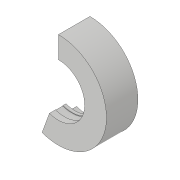
# Autodesk Inventor part: 00_Adapter_M8_Fluorescentfilter_Cellphone
Saved by Autodesk Inventor 2019 (Build 230136000, 136)
## iProperties
Created: 2019-06-13
Part Number: 00_Adapter_M8_Fluorescentfilter_Cellphone
Material: Generic
Document SubType Name: Modeling
Designer: diederichbenedict
Density: 1 g/cm^3
Appearance: Default
Author: diederichbenedict
Autodesk Inventor part; units mm, degrees
ref_plane "YZ Plane" through (0, 0, 0) normal (1, 0, 0) x (0, 1, 0)
ref_plane "XZ Plane" through (0, 0, 0) normal (0, 1, 0) x (-1, 0, 0)
ref_plane "XY Plane" through (0, 0, 0) normal (0, 0, 1) x (1, 0, 0)
sketch "Sketch1" plane through (0, 0, 0) normal (1, 0, 0) x (0, 1, 0)
  line L0 (0, 0) -> (8.75, 0) construction
  line L1 (8.75, 0) -> (8.75, -2)
  line L2 (8.75, -2) -> (8.9374, -2)
  line L3 (8.9374, -2) -> (8.9374, -4.5)
  line L4 (8.9374, -4.5) -> (8.75, -4.5)
  line L5 (8.75, -4.5) -> (8.75, -5.5)
  line L6 (8.75, -5.5) -> (13, -5.5)
  line L7 (13, -5.5) -> (13, -10.5)
  line L8 (13, -10.5) -> (16, -10.5)
  line L9 (16, -10.5) -> (16, 0)
  line L10 (16, 0) -> (8.75, 0)
  line L11 (0, 0) -> (0, -14.519)
  dimension "d0" = 8.75
  dimension "d1" = 2
  dimension "d2" = 2.5
  dimension "d3" = 1
  dimension "d4" = 5
  dimension "d5" = 13
  dimension "d8" = 16
  constraints: 24 end point, 8 perpendicular, 2 point on line, 2 vertical, 1 horizontal
  measures "d0" distance of L0.start L0.end
  measures "d1" distance of L0.end L1.end
  measures "d2" distance of L2.end L3.end
  measures "d3" distance of L4.end L5.end
  measures "d4" distance of L6.end L7.end
  measures "d5" distance between parallel lines of L7 L11
  measures "d8" distance between parallel lines of L9 L11
revolve "Revolution1" add sketch "Sketch1" angle 200 about axis through (0, 0, 0) along (0, 0, -1)
body "Solid1"
